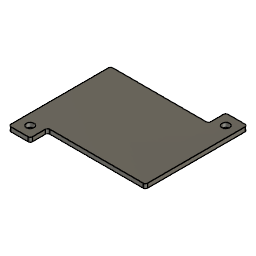
Battery Cover (Autodesk Fusion 360 design; units mm, degrees)
Autodesk Fusion 360 part; units mm, degrees
sketch "Sketch1" plane through (0, 0, 0) normal (0, 0, 1) x (1, 0, 0)
  line L0 (0, 0) -> (55, 0)
  line L1 (55, 0) -> (55, 55)
  line L2 (55, 55) -> (0, 55)
  line L3 (0, 55) -> (0, 0)
  line L4 (55, 55) -> (45, 55)
  line L5 (45, 55) -> (45, 47)
  line L6 (45, 47) -> (55, 47)
  line L7 (55, 47) -> (55, 55)
  line L8 (0, 0) -> (10, 0)
  line L9 (10, 0) -> (10, 8)
  line L10 (10, 8) -> (0, 8)
  line L11 (0, 8) -> (0, 0)
  line L12 (0, 8) -> (55, 8)
  line L13 (55, 8) -> (55, 47)
  line L14 (55, 47) -> (0, 47)
  line L15 (0, 47) -> (0, 8)
  circle A0 centre (5, 5) radius 1.75
  circle A1 centre (50, 50) radius 1.75
  line L16 (0, 10) -> (55, 10)
  line L17 (55, 10) -> (55, 45)
  line L18 (55, 45) -> (0, 45)
  line L19 (0, 45) -> (0, 10)
  dimension "d1" = 55
  dimension "d7" = 3.5
  dimension "d8" = 3.5
  dimension "d9" = 5
  dimension "d11" = 5
  dimension "d47" = 39
  dimension "d48" = 55
  dimension "d49" = 35
  dimension "d50" = 2
  dimension "d53" = 5
  dimension "d54" = 5
  dimension "d55" = 8
  dimension "d56" = 8
  dimension "d57" = 10
  dimension "d58" = 10
  constraint horizontal L0
  constraint vertical L1
  constraint horizontal L2
  constraint vertical L3
  constraint coincident L0.start L3.end
  constraint horizontal L4
  constraint vertical L5
  constraint horizontal L6
  constraint vertical L7
  constraint horizontal L8
  constraint vertical L9
  constraint horizontal L10
  constraint vertical L11
  constraint horizontal L12
  constraint vertical L13
  constraint horizontal L14
  constraint vertical L15
  constraint horizontal L16
  constraint vertical L17
  constraint horizontal L18
  constraint vertical L19
  constraint coincident L3 L16.start
  measures "d1" distance of L0.start L0.end
  measures "d7" diameter of A0
  measures "d8" diameter of A1
  measures "d9" distance of L9 A0.centre
  measures "d11" distance of L7 A1.centre
  measures "d47" distance of L12 L14
  measures "d48" distance of L16.start L16.end
  measures "d49" distance of L16.start L18.end
  measures "d50" distance of L12 L16
  measures "d53" distance of A1.centre L18
  measures "d54" distance of A0.centre L16
  measures "d55" distance of L2 L14
  measures "d56" distance of L8 L12
  measures "d57" distance of L1 L5
  measures "d58" distance of L9 L11
extrude "Extrude1" add sketch "Sketch1" along normal blind 2 contours L0 L3 L8 L9 L10 L11 L12 | L1 L3 L10 L12 L13 L15 L16 | L1 L3 L13 L15 L16 L17 L18 L19 | L1 L3 L6 L13 L14 L15 L18 | L1 L2 L4 L5 L6 L7 L14
sketch "Sketch2" plane through (0, 0, 2) normal (0, 0, 1) x (-1, 0, 0)
  circle A0 centre (-50, -50) radius 1.75
  circle A1 centre (-5, -5) radius 1.75
  line L0 (0, -47) -> (0, 0)
  line L1 (0, 0) -> (-10, 0)
  line L2 (-10, 0) -> (-10, -8)
  line L3 (-10, -8) -> (-55, -8)
  line L4 (-55, -8) -> (-55, -55)
  line L5 (-55, -55) -> (-45, -55)
  line L6 (-45, -55) -> (-45, -47)
  line L7 (-45, -47) -> (0, -47)
  circle A2 centre (-5, -5) radius 1.875
  circle A3 centre (-50, -50) radius 1.875
  line L8 (-4.0912, -23.3213) -> (-51.331, -24.5146) construction
  line L9 (-51.331, -24.5146) -> (-51.1199, -32.872) construction
  line L10 (-51.1199, -32.872) -> (-3.8801, -31.6787) construction
  line L11 (-3.8801, -31.6787) -> (-4.0912, -23.3213) construction
  line L12 (0, -47) -> (0, -8)
  line L13 (0, -8) -> (-55, -8)
  dimension "d15" = 3.75
  dimension "d40" = 5
  dimension "d41" = 27.5
  dimension "d42" = 19.5
  constraint concentric A1 A2
  constraint concentric A0 A3
  measures "d15" diameter of A3
hole "Hole1" at (50, 50, 2) direction (0, 0, -1) diameter 3.5 depth 2 tip angle 118
hole "Hole2" at (5, 5, 2) direction (0, 0, -1) diameter 3.5 depth 2 tip angle 118
fillet "Fillet1" radius 1 1 edges at (0, 47, 1)
fillet "Fillet2" radius 1 1 edges at (45, 55, 1)
fillet "Fillet3" radius 1 1 edges at (45, 47, 1)
fillet "Fillet4" radius 1 1 edges at (55, 55, 1)
fillet "Fillet5" radius 1 2 edges at (0, 0, 1) (10, 0, 1)
fillet "Fillet6" radius 1 1 edges at (10, 8, 1)
fillet "Fillet7" radius 1 1 edges at (55, 8, 1)
emboss "Emboss1" [suppressed]
